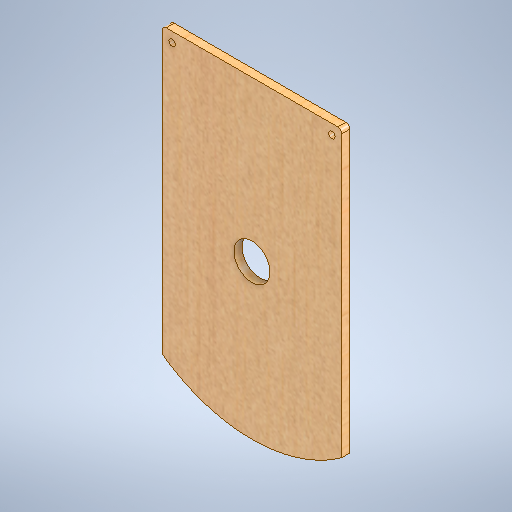
# Autodesk Inventor part: onering_plate_test_nomotor
Saved by Autodesk Inventor 2025.1 (Build 291241000, 241)
## iProperties
Created: 2024-11-11
Part Number: onering_plate_test_nomotor
Material: 一般
Document SubType Name: Modeling
Designer: yuki0520
Density: 1 g/cm^3
Appearance: イエロー パイン材 - 硬質 塗装 抑えた光沢
Author: yuki0520
Autodesk Inventor part; units mm, degrees
ref_plane "YZ Plane" through (0, 0, 0) normal (1, 0, 0) x (0, 1, 0)
ref_plane "XZ Plane" through (0, 0, 0) normal (0, 1, 0) x (-1, 0, 0)
ref_plane "XY Plane" through (0, 0, 0) normal (0, 0, 1) x (1, 0, 0)
derived "zzz_yoko3.ipt"
sketch "スケッチ1" plane through (0, 0, 0) normal (0, 0, 1) x (1, 0, 0)
  circle A0 centre (0, 0) radius 77
  line L0 (45, -80) -> (-45, -80)
  line L1 (-45, -80) -> (-45, 80)
  line L2 (-45, 80) -> (45, 80)
  line L3 (45, 80) -> (45, -80)
  line L4 (45, -80) -> (-45, 80) construction
  line L5 (-45, -80) -> (45, 80) construction
  circle A1 centre (197, 0) radius 120
  circle A2 centre (0, 197) radius 120
  line L6 (-45, 0) -> (45, 0)
  arc A3 (317, 0) -> (0, 317) centre (0, 0) ccw
  line L7 (0, 0) -> (0, 317) construction
  line L8 (0, 0) -> (317, 0) construction
  line L9 (0, 317) -> (0, 0)
  line L10 (317, 0) -> (0, 0)
  line L11 (335.5, -103) -> (317, -103)
  line L12 (317, -103) -> (317, 103)
  line L13 (317, 103) -> (335.5, 103)
  line L14 (335.5, 103) -> (335.5, -103)
  line L15 (335.5, -103) -> (317, 103) construction
  line L16 (317, -103) -> (335.5, 103) construction
  line L17 (-103, 317) -> (-103, 335.5)
  line L18 (-103, 335.5) -> (103, 335.5)
  line L19 (103, 335.5) -> (103, 317)
  line L20 (103, 317) -> (-103, 317)
  line L21 (-35, -80) -> (-35, 345.5)
  line L22 (0, 317) -> (0, 347)
  line L23 (317, 0) -> (347, 0)
  line L24 (227.3, -103) -> (166.7, -103)
  line L25 (166.7, -103) -> (166.7, 103)
  line L26 (166.7, 103) -> (227.3, 103)
  line L27 (227.3, 103) -> (227.3, -103)
  line L28 (227.3, -103) -> (166.7, 103) construction
  line L29 (166.7, -103) -> (227.3, 103) construction
  line L30 (197, 103) -> (197, -103)
  line L31 (-45, 94) -> (355, 94)
  line L32 (-45, -94) -> (355, -94)
  line L33 (35, -80) -> (35, 345.5)
  line L34 (-113, 335.5) -> (113, 335.5)
  line L35 (113, 335.5) -> (113, 345.5)
  line L36 (113, 345.5) -> (-113, 345.5)
  line L37 (-113, 345.5) -> (-113, 335.5)
  line L38 (35, 345.5) -> (45, 345.5)
  line L39 (45, 345.5) -> (45, 355.5)
  line L40 (45, 355.5) -> (35, 355.5)
  line L41 (35, 355.5) -> (35, 345.5)
  circle A4 centre (0, 0) radius 9
  line L42 (335.5, 113) -> (345.5, 113)
  line L43 (345.5, 113) -> (345.5, -107)
  line L44 (345.5, -107) -> (335.5, -107)
  line L45 (335.5, -107) -> (335.5, 113)
  arc A5 (345.5, 113) -> (113, 345.5) centre (0, 0) ccw
  line L46 (103, 335.5) -> (103, 299.7999)
  line L47 (335.5, 103) -> (299.7999, 103)
  line L48 (113, 345.5) -> (113, 296.1756)
  line L49 (-40, -80) -> (-30, -80)
  line L50 (-30, -80) -> (-30, 355.5)
  line L51 (-30, 355.5) -> (-40, 355.5)
  line L52 (-40, 345.5) -> (-40, -80)
  line L53 (-45, -75) -> (345.5, -75)
  line L54 (345.5, -75) -> (345.5, -65)
  line L55 (345.5, -65) -> (-45, -65)
  line L56 (-45, -65) -> (-45, -75)
  line L57 (-40, 345.5) -> (-50, 345.5)
  line L58 (-30, 355.5) -> (-40, 355.5)
  line L59 (-50, 345.5) -> (-40, 345.5)
  line L60 (-40, 345.5) -> (-40, 355.5)
  line L61 (-40, 355.5) -> (-50, 355.5)
  line L62 (-50, 355.5) -> (-50, 345.5)
  line L63 (-45, 80) -> (-55, 80)
  line L64 (-55, 80) -> (-55, 70)
  line L65 (-55, 70) -> (-45, 70)
  line L66 (-45, 70) -> (-45, 80)
  line L67 (-45, -80) -> (-55, -80)
  line L68 (75, -65) -> (75, -75)
  line L69 (-45, -80) -> (345.5, -80)
  line L70 (-45, -65) -> (-70, -65)
  line L71 (-70, -65) -> (-70, -75)
  line L72 (-70, -75) -> (-45, -75)
  line L73 (-45, -75) -> (-45, -65)
  line L74 (345.5, -75) -> (370.5, -75)
  line L75 (370.5, -75) -> (370.5, -65)
  line L76 (370.5, -65) -> (345.5, -65)
  line L77 (345.5, -65) -> (345.5, -75)
  line L78 (-103, 335.5) -> (-103, 345.5)
  point P0 (326.25, 0)
  point P1 (0, 335.5)
  point P2 (197, 0)
extrude "押し出し1" add sketch "スケッチ1" along normal blind 4 contours L3 L6 L33 A0 | A0 L33 L2 L3 | L3 L55 A0 | A0 L55 L33 L6 L3 | L33 L6 A4 L9 A0 | A0 A2 L2 L33 | L55 L3 L53 L33 A0 | A0 L33 L55 | L33 L55 L50 L6 A4 | L9 A4 L6 L50 A0 | A0 L50 L2 A2 | L9 L2 A2 | A2 L2 L9 | L33 L53 A0 | A0 L53 L50 L55 L33 | L3 L0 L33 L53 | L50 L6 L21 A0 | A0 L21 L2 L50 | L53 L33 L0 L50 A0 | A0 L53 | L55 L21 L6 L50 | L50 A0 L21 L55 | L21 L6 L52 A0 | A0 L52 L2 L21 | L53 L50 A0 | L50 L53 L21 A0 | L55 L52 L6 L21 | L21 A0 L52 L55 | L52 L6 L1 A0 | A0 L1 L2 L52 | L50 L0 L21 L53 | L21 L53 L52 A0 | L55 A0 L1 L6 L52 | L52 A0 L55 | L21 L0 L52 L53 | L52 L53 L1 L55 A0 | L55 L1 A0 | L52 L0 L1 L53
sketch "スケッチ2" plane through (-45, -80, 4) normal (0, 0, 1) x (1, 0, 0)
  line L0 (0, 160) -> (0, 0) projected
  line L1 (0, 0) -> (90, 0) projected
  line L2 (90, 0) -> (90, 160) projected
  line L3 (90, 160) -> (0, 160) projected
  circle A0 centre (45, 80) radius 9 projected
  line L4 (5, 5) -> (5, 155)
  line L5 (5, 155) -> (85, 155)
  line L6 (85, 155) -> (85, 5)
  line L7 (85, 5) -> (5, 5)
  point P0 (5, 150.5)
  point P1 (85, 150.5)
  dimension "d3" = 5
  constraints: 8 end point, 4 coincident, 2 point on line, 3 other
  measures "d3" distance between parallel lines of L0 L4
hole "穴1" at (-40, 75, 4) at (40, 75, 4) at (-40, -75, 4) at (40, -75, 4) direction (0, 0, -1) diameter 3.2 end through all
fillet "フィレット1" radius 2 4 edges at (-45, 80, 2) (45, 80, 2) (45, -80, 2) (-45, -80, 2)
sketch "スケッチ3" plane through (-43, -80, 4) normal (0, 0, 1) x (1, 0, 0)
  circle A0 centre (43, 80) radius 77
  circle A1 centre (83, 5) radius 1.6 projected
  circle A2 centre (3, 5) radius 1.6 projected
  circle A3 centre (83, 155) radius 1.6 projected
  circle A4 centre (3, 155) radius 1.6 projected
  arc A5 (-2, 2) -> (0, 0) centre (0, 2) ccw projected
  line L0 (0, 0) -> (86, 0) projected
  arc A6 (86, 0) -> (88, 2) centre (86, 2) ccw projected
  line L1 (88, 2) -> (88, 158) projected
  arc A7 (88, 158) -> (86, 160) centre (86, 158) ccw projected
  line L2 (86, 160) -> (0, 160) projected
  arc A8 (0, 160) -> (-2, 158) centre (0, 158) ccw projected
  line L3 (-2, 158) -> (-2, 2) projected
  circle A9 centre (43, 80) radius 9 projected
  point P0 (88, 17.518)
  point P1 (-2, 17.518)
  dimension "d15" = 154
  constraints: 1 centre point, 1 coincident
  measures "d15" diameter of A0
extrude "押し出し2" cut sketch "スケッチ3" against normal blind 10 contours L1 A6 L0 A5 L3 A0
